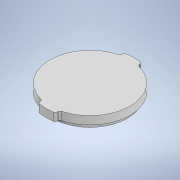
# Autodesk Inventor part: HSI cap
Saved by Autodesk Inventor 2022 (Build 260153000, 153)
## iProperties
Created: 2022-03-31
Part Number: HSI cap
Material: Generic
Document SubType Name: Modeling
Designer: RNG3nius
Density: 1 g/cm^3
Appearance: Default
Author: RNG3nius
Autodesk Inventor part; units mm, degrees
ref_plane "YZ Plane" through (0, 0, 0) normal (1, 0, 0) x (0, 1, 0)
ref_plane "XZ Plane" through (0, 0, 0) normal (0, 1, 0) x (-1, 0, 0)
ref_plane "XY Plane" through (0, 0, 0) normal (0, 0, 1) x (1, 0, 0)
sketch "Sketch1" plane through (0, 0, 0) normal (0, 1, 0) x (-1, 0, 0)
  circle A0 centre (0, 0) radius 26.725
  dimension "d0" = 53.45
  constraints: 1 centre point, 1 coincident
  measures "d0" diameter of A0
extrude "Extrusion1" add sketch "Sketch1" along normal blind 3
sketch "Sketch2" plane through (0, 3, 0) normal (0, 1, 0) x (1, 0, 0)
  circle A0 centre (0, 0) radius 28.8
  dimension "d3" = 57.6
  constraints: 1 centre point, 1 coincident
  measures "d3" diameter of A0
extrude "Extrusion2" add sketch "Sketch2" along normal blind 5.8
sketch "Sketch4" plane through (0, 8.8, 0) normal (0, 1, 0) x (1, 0, 0)
  circle A0 centre (0, 0) radius 31.65
  circle A1 centre (0, 0) radius 28.8
  circle A2 centre (0, 0) radius 28.8 projected
  line L0 (6.3178, -28.0985) -> (-6.3178, -28.0985)
  line L1 (-6.3178, -28.0985) -> (-6.3178, -31.013)
  line L2 (6.3178, -28.0985) -> (6.3178, -31.013)
  line L3 (-6.3178, 28.0985) -> (6.3178, 28.0985)
  line L4 (6.3178, 28.0985) -> (6.3178, 31.013)
  line L5 (-6.3178, 28.0985) -> (-6.3178, 31.013)
  dimension "d13" = 63.3
  dimension "d16" = 360
  dimension "d18" = 56.197
  constraints: 12 end point, 4 point on circle, 2 coincident, 2 parallel, 2 point on line, 1 centre point, 1 horizontal, 1 perpendicular, 20 other
  measures "d13" diameter of A0
  measures "d18" distance between parallel lines of L3 L0
extrude "Extrusion3" add sketch "Sketch4" against normal up to surface (5.8 mm away) contours L4 A1 L5 A0 | A0 L1 A1 L2
fillet "Fillet1" radius 1.4575 8 edges at (-6.3178, 5.9, 28.0985) (-6.3178, 5.9, 31.013) (6.3178, 5.9, 31.013) (6.3178, 5.9, 28.0985) (6.3178, 5.9, -28.0985) (6.3178, 5.9, -31.013) (-6.3178, 5.9, -28.0985) (-6.3178, 5.9, -31.013)
body "Solid1"
